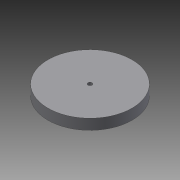
# Autodesk Inventor part: Wheel
Saved by Autodesk Inventor 2015 (Build 190159000, 159)
## iProperties
Created: 2014-07-26
Part Number: Wheel
Material: Generic
Document SubType Name: Modeling
Designer: karl
Density: 1 g/cm^3
Appearance: Default
Author: karl
Autodesk Inventor part; units mm, degrees
ref_plane "YZ Plane" through (0, 0, 0) normal (1, 0, 0) x (0, 1, 0)
ref_plane "XZ Plane" through (0, 0, 0) normal (0, 1, 0) x (-1, 0, 0)
ref_plane "XY Plane" through (0, 0, 0) normal (0, 0, 1) x (1, 0, 0)
sketch "Sketch1" plane through (0, 0, 0) normal (0, 0, 1) x (1, 0, 0)
  circle A0 centre (0, 0) radius 30
  circle A1 centre (0, 0) radius 2
  dimension "d0" = 60
  dimension "d1" = 4
  constraints: 2 centre point, 2 coincident
  measures "d0" diameter of A0
  measures "d1" diameter of A1
extrude "Extrusion1" add sketch "Sketch1" along normal blind 10
sketch "Sketch2" plane through (0, 0, 10) normal (0, 0, 1) x (1, 0, 0)
  circle A0 centre (0, 0) radius 7.5
  circle A1 centre (0, 0) radius 2 projected
  circle A2 centre (0, 0) radius 27.5
  line L0 (-0.75, 7.4624) -> (-3, 27.3359)
  line L1 (0.75, 7.4624) -> (3, 27.3359)
  line L2 (-3, 27.3359) -> (3, 27.3359) construction
  line L3 (-0.75, 7.4624) -> (0.75, 7.4624) construction
  point P0 (0, 27.3359)
  dimension "d4" = 15
  dimension "d5" = 55
  dimension "d6" = 1.5
  dimension "d7" = 6
  constraints: 8 end point, 4 point on circle, 2 centre point, 2 coincident, 1 horizontal, 1 midpoint, 1 parallel, 1 vertical alignment
  measures "d4" diameter of A0
  measures "d5" diameter of A2
  measures "d6" distance of L0.start L1.start
  measures "d7" distance of L0.end L1.end
extrude "Extrusion2" cut sketch "Sketch2" against normal blind 10 contours A0 L0 A2 L1 picked at (-0.0835, 20.8198)
pattern_circular "Circular Pattern1" count 15 over 360 about axis through (0, 0, 0) along (0, 0, 1) of "Extrusion2"
sketch "Sketch3" plane through (0, 0, 10) normal (0, 0, 1) x (1, 0, 0)
  circle A0 centre (0, 0) radius 6
  circle A1 centre (0, 0) radius 27.5
  dimension "d13" = 55
  dimension "d14" = 12
  constraints: 2 centre point, 2 coincident
  measures "d13" diameter of A1
  measures "d14" diameter of A0
extrude "Extrusion3" cut sketch "Sketch3" against normal blind 3
fillet "Fillet1" radius 2 1 edges at (-6, 0, 7)
ref_plane "Work Plane1" through (0, 0, 5) normal (0, 0, 1) x (1, 0, 0)
mirror "Mirror1" about plane through (0, 0, 5) normal (0, 0, 1) of "Fillet1", "Extrusion3"
body "Solid1"
